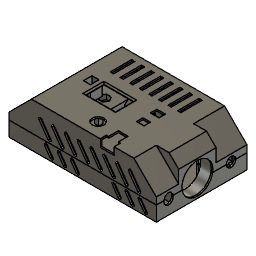
Arduino_Spot_Welder_V4_Case (Autodesk Fusion 360 design; units mm, degrees)
Autodesk Fusion 360 part; units mm, degrees
note: some values were not read from the file. Chosen so that the rebuilt part matches the saved one: a direction; which face or edge a step refers to; a side. Set by a fixed rule: which sketch regions a step uses.
(part 1 of 2)
sketch "Skizze1" plane through (0, 0, 0) normal (0, 1, 0) x (1, 0, 0)
  line L0 (-67.5, -41) -> (67.5, -41)
  line L1 (67.5, -41) -> (67.5, 41)
  line L2 (67.5, 41) -> (-67.5, 41)
  line L3 (-67.5, 41) -> (-67.5, -41)
  line L4 (1.75, 0) -> (22.5, 0)
  line L5 (0, -1.75) -> (0, -22.5)
  dimension "d1" = 82
  dimension "d2" = 135
  constraint horizontal L0
  constraint vertical L1
  constraint horizontal L2
  constraint vertical L3
  constraint symmetric L0 L2 L4
  constraint symmetric L1 L3 L5
  measures "d1" distance of L0.start L2.end
  measures "d2" distance of L0.start L0.end
extrude "Extrusion1" add sketch "Skizze1" along normal blind 1.5 makes body 1
sketch "Skizze2" plane through (0, 1.5, 0) normal (0, 1, 0) x (-1, 0, 0)
  line L0 (67.5, -41) -> (67.5, 41)
  line L1 (67.5, 41) -> (-67.5, 41)
  line L2 (-67.5, 41) -> (-67.5, -41)
  line L3 (-67.5, -41) -> (67.5, -41)
  line L4 (38.5, 39) -> (-38.5, 39)
  line L5 (-38.5, 39) -> (-38.5, -11)
  line L6 (-38.5, -11) -> (38.5, -11)
  line L7 (38.5, -11) -> (38.5, 39)
  line L8 (-1.75, 0) -> (-22.5, 0)
  line L9 (0, 1.75) -> (0, 22.5)
  circle A0 centre (35.5, 36) radius 1.65
  circle A1 centre (-35.5, -8) radius 1.65
  line L10 (38.5, 39) -> (32.5, 39)
  line L11 (32.5, 39) -> (32.5, 33)
  line L12 (32.5, 33) -> (38.5, 33)
  line L13 (38.5, 33) -> (38.5, 39)
  line L14 (-38.5, -11) -> (-32.5, -11)
  line L15 (-32.5, -11) -> (-32.5, -5)
  line L16 (-32.5, -5) -> (-38.5, -5)
  line L17 (-38.5, -5) -> (-38.5, -11)
  line L18 (38.5, -11) -> (34.5, -11)
  line L19 (34.5, -11) -> (34.5, -7)
  line L20 (34.5, -7) -> (38.5, -7)
  line L21 (38.5, -7) -> (38.5, -11)
  line L22 (-38.5, 39) -> (-34.5, 39)
  line L23 (-34.5, 39) -> (-34.5, 35)
  line L24 (-34.5, 35) -> (-38.5, 35)
  line L25 (-38.5, 35) -> (-38.5, 39)
  dimension "d5" = 77
  dimension "d6" = 50
  dimension "d7" = 2
  dimension "d8" = 3.3
  dimension "d9" = 3.3
  dimension "d10" = 3
  dimension "d11" = 3
  dimension "d12" = 3
  dimension "d13" = 3
  dimension "d14" = 6
  dimension "d15" = 6
  dimension "d16" = 6
  dimension "d17" = 6
  dimension "d302" = 4
  dimension "d303" = 4
  dimension "d304" = 4
  dimension "d305" = 4
  constraint horizontal L4
  constraint vertical L5
  constraint horizontal L6
  constraint vertical L7
  constraint symmetric L5 L7 L9
  constraint horizontal L10
  constraint vertical L11
  constraint horizontal L12
  constraint vertical L13
  constraint horizontal L14
  constraint vertical L15
  constraint horizontal L16
  constraint vertical L17
  constraint horizontal L18
  constraint vertical L19
  constraint horizontal L20
  constraint vertical L21
  constraint horizontal L22
  constraint vertical L23
  constraint horizontal L24
  constraint vertical L25
  measures "d5" distance of L4.start L4.end
  measures "d6" distance of L4.start L6.end
  measures "d7" distance of L1 L4
  measures "d8" diameter of A0
  measures "d9" diameter of A1
  measures "d10" distance of L4 A0.centre
  measures "d11" distance of L7 A0.centre
  measures "d12" distance of L5 A1.centre
  measures "d13" distance of L6 A1.centre
  measures "d14" distance of L4.start L10.end
  measures "d15" distance of L4.start L12.end
  measures "d16" distance of L5.end L14.end
  measures "d17" distance of L5.end L16.end
  measures "d302" distance of L6.end L18.end
  measures "d303" distance of L6.end L20.end
  measures "d304" distance of L4.end L22.end
  measures "d305" distance of L4.end L24.end
extrude "Extrusion2" add sketch "Skizze2" along normal blind 5.5 contours L4 L7 L10 L11 L12 L13 | L5 L6 L14 L15 L16 L17 bodies 1
extrude "Extrusion3" add 2 faces at (-35.3776, 1.5, 36.5362) (35.9032, 1.5, -8.3741) along direction (0, 1, 0) blind 2 on bodies 1 bodies 1
extrude "Extrusion57" add sketch "Skizze2" along normal blind 8 contours L4 L5 L22 L23 L24 L25 | L6 L7 L18 L19 L20 L21 bodies 1
sketch "Skizze3" plane through (0, 1.5, 0) normal (0, 1, 0) x (-1, 0, 0)
  line L0 (38.5, 33) -> (32.5, 33)
  line L1 (32.5, 33) -> (32.5, 39)
  line L2 (32.5, 39) -> (38.5, 39)
  line L3 (38.5, 39) -> (38.5, 33)
  line L4 (67.5, -41) -> (67.5, 41)
  line L5 (67.5, 41) -> (-67.5, 41)
  line L6 (-67.5, 41) -> (-67.5, -41)
  line L7 (-67.5, -41) -> (67.5, -41)
  line L8 (-38.5, -5) -> (-32.5, -5)
  line L9 (-32.5, -5) -> (-32.5, -11)
  line L10 (-32.5, -11) -> (-38.5, -11)
  line L11 (-38.5, -11) -> (-38.5, -5)
  line L12 (61, -16) -> (-25, -16)
  line L13 (-25, -16) -> (-25, -39)
  line L14 (-25, -39) -> (61, -39)
  line L15 (61, -39) -> (61, -16)
  line L16 (0, 1.75) -> (0, 22.5)
  line L17 (-1.75, 0) -> (-22.5, 0)
  line L18 (35.5, -39) -> (0.5, -39)
  line L19 (0.5, -39) -> (0.5, -16)
  line L20 (0.5, -16) -> (35.5, -16)
  line L21 (35.5, -16) -> (35.5, -39)
  line L22 (-38.5, 35) -> (-38.5, 39)
  line L23 (-38.5, 39) -> (-34.5, 39)
  line L24 (-34.5, 39) -> (-34.5, 35)
  line L25 (-34.5, 35) -> (-38.5, 35)
  line L26 (38.5, -7) -> (38.5, -11)
  line L27 (38.5, -11) -> (34.5, -11)
  line L28 (34.5, -11) -> (34.5, -7)
  line L29 (34.5, -7) -> (38.5, -7)
  dimension "d22" = 86
  dimension "d23" = 23
  dimension "d24" = 2
  dimension "d25" = 35
  dimension "d369" = 25.5
  dimension "d370" = 6.5
  constraint horizontal L12
  constraint vertical L13
  constraint horizontal L14
  constraint vertical L15
  constraint horizontal L18
  constraint vertical L19
  constraint horizontal L20
  constraint vertical L21
  constraint coincident L14 L18.start
  constraint collinear L12 L20
  measures "d22" distance of L12.start L12.end
  measures "d23" distance of L12.start L14.end
  measures "d24" distance of L7 L14
  measures "d25" distance of L18.start L18.end
  measures "d229" distance of L20.end
  measures "d369" distance of L13 L19
  measures "d370" distance of L4 L15
extrude "Extrusion4" add sketch "Skizze3" along normal blind 5 contours L12 L14 L15 L21 | L12 L13 L14 L19 bodies 1
sketch "Skizze4" plane through (0, 6.5, 0) normal (0, 1, 0) x (-1, 0, 0)
  line L0 (35.5, -16) -> (35.5, -39)
  line L1 (35.5, -39) -> (61, -39)
  line L2 (61, -39) -> (61, -16)
  line L3 (61, -16) -> (35.5, -16)
  line L4 (51.8383, -31.55) -> (54.1765, -27.5)
  line L5 (54.1765, -27.5) -> (51.8383, -23.45)
  line L6 (51.8383, -23.45) -> (47.1617, -23.45)
  line L7 (47.1617, -23.45) -> (44.8235, -27.5)
  line L8 (44.8235, -27.5) -> (47.1617, -31.55)
  line L9 (47.1617, -31.55) -> (51.8383, -31.55)
  line L10 (0, 1.75) -> (0, 22.5)
  circle A0 centre (49.5, -27.5) radius 2.6
  circle A1 centre (-13.5, -28) radius 2.6
  line L11 (-11.1617, -32.05) -> (-8.8235, -28)
  line L12 (-8.8235, -28) -> (-11.1617, -23.95)
  line L13 (-11.1617, -23.95) -> (-15.8383, -23.95)
  line L14 (-15.8383, -23.95) -> (-18.1765, -28)
  line L15 (-18.1765, -28) -> (-15.8383, -32.05)
  line L16 (-15.8383, -32.05) -> (-11.1617, -32.05)
  line L17 (0.5, -39) -> (0.5, -16)
  line L18 (-25, -39) -> (0.5, -39)
  point P0 (49.5, -27.5)
  point P1 (-13.5, -28)
  dimension "d28" = 4.05
  dimension "d29" = 11.5
  dimension "d31" = 14
  dimension "d35" = 5.2
  dimension "d371" = 5.2
  dimension "d372" = 4.05
  dimension "d373" = 14
  dimension "d374" = 11
  constraint parallel L1 L9
  constraint coincident P0 A0.centre
  constraint coincident P1 A1.centre
  constraint parallel L16 L18
  measures "d28" distance of P0 L9
  measures "d29" distance of L1 P0
  measures "d31" distance of L0 P0
  measures "d35" diameter of A0
  measures "d371" diameter of A1
  measures "d372" distance of P1 L16
  measures "d373" distance of P1 L17
  measures "d374" distance of P1 L18
extrude "Extrusion5" cut sketch "Skizze4" against normal blind 4.5 contours L4 L5 L6 L7 L8 L9 | A0 | A1 | L11 L12 L13 L14 L15 L16 bodies 1
extrude "Extrusion6" cut sketch "Skizze4" against normal up to surface (5.5 mm away) contours A0 | A1 bodies 1
sketch "Skizze6" plane through (0, 0, 0) normal (0, -1, 0) x (1, 0, 0)
  line L0 (-67.5, 41) -> (-67.5, -41)
  line L1 (-67.5, -41) -> (67.5, -41)
  line L2 (67.5, -41) -> (67.5, 41)
  line L3 (67.5, 41) -> (-67.5, 41)
  line L4 (-69, -42.5) -> (69, -42.5)
  line L5 (69, -42.5) -> (69, 42.5)
  line L6 (69, 42.5) -> (-69, 42.5)
  line L7 (-69, 42.5) -> (-69, -42.5)
  dimension "d38" = 1.5
  dimension "d39" = 1.5
  dimension "d40" = 1.5
  dimension "d41" = 1.5
  constraint horizontal L4
  constraint vertical L5
  constraint horizontal L6
  constraint vertical L7
  measures "d38" distance of L0 L7
  measures "d39" distance of L2 L5
  measures "d40" distance of L3 L6
  measures "d41" distance of L1 L4
extrude "Extrusion7" add sketch "Skizze6" against normal blind 14 bodies 1
extrude "Extrusion69" add 1 faces at (-36.5, 3.3333, 39) along direction (0, 0, 1) up to surface (2 mm away) on bodies 1 bodies 1
extrude "Extrusion71" add 1 faces at (35.8333, 4.1667, 39) along direction (0, 0, 1) up to surface (2 mm away) on bodies 1 bodies 1
sketch "Skizze58" plane through (0, 0, -11) normal (0, 0, -1) x (-1, 0, 0)
  line L0 (34.5, 1.5) -> (38.5, 1.5)
  line L1 (38.5, 1.5) -> (38.5, 9.5)
  line L2 (38.5, 9.5) -> (34.5, 9.5)
  line L3 (34.5, 9.5) -> (34.5, 1.5)
  line L4 (61, 1.5) -> (35.5, 1.5)
  line L5 (35.5, 1.5) -> (35.5, 6.5)
  line L6 (35.5, 6.5) -> (61, 6.5)
  line L7 (61, 6.5) -> (61, 1.5)
extrude "Extrusion73" add sketch "Skizze58" along normal up to surface (5 mm away) contours L0 L1 L4 L5 L6 bodies 1
sketch "Skizze7" plane through (-69, 0, 0) normal (-1, 0, 0) x (0, 0, 1)
  line L0 (-42.5, 0) -> (42.5, 0)
  line L1 (42.5, 0) -> (42.5, 14)
  line L2 (42.5, 14) -> (-42.5, 14)
  line L3 (-42.5, 14) -> (-42.5, 0)
  circle A0 centre (-27.5, 14) radius 4.5
  dimension "d44" = 9
  dimension "d46" = 15
  constraint coincident L2 A0.centre
  measures "d44" diameter of A0
  measures "d46" distance of L3 A0.centre
extrude "Extrusion8" cut sketch "Skizze7" against normal blind 138 contours L2 A0 picked at (-26.2064, 11.6926) bodies 1
sketch "Skizze8" plane through (-69, 0, 0) normal (-1, 0, 0) x (0, 0, 1)
  arc A0 (-32, 14) -> (-23, 14) centre (-27.5, 14) ccw
  line L0 (-32, 14) -> (-42.5, 14)
  line L1 (-42.5, 14) -> (-42.5, 0)
  line L2 (-42.5, 0) -> (42.5, 0)
  line L3 (42.5, 0) -> (42.5, 14)
  line L4 (42.5, 14) -> (-23, 14)
  circle A1 centre (-2.5, 14) radius 4.5
  dimension "d49" = 9
  dimension "d51" = 45
  constraint coincident L4 A1.centre
  measures "d49" diameter of A1
  measures "d51" distance of L3 A1.centre
extrude "Extrusion9" cut sketch "Skizze8" against normal blind 2 contours L4 A1 picked at (-1, 11.9595) bodies 1
sketch "Skizze9" plane through (69, 0, 0) normal (1, 0, 0) x (0, 0, -1)
  arc A0 (23, 14) -> (32, 14) centre (27.5, 14) ccw
  line L0 (23, 14) -> (-42.5, 14)
  line L1 (-42.5, 14) -> (-42.5, 0)
  line L2 (-42.5, 0) -> (42.5, 0)
  line L3 (42.5, 0) -> (42.5, 14)
  line L4 (42.5, 14) -> (32, 14)
  circle A1 centre (-31, 14) radius 4.25
  dimension "d54" = 8.5
  dimension "d55" = 11.5
  constraint coincident L0 A1.centre
  measures "d54" diameter of A1
  measures "d55" distance of L1 A1.centre
extrude "Extrusion10" cut sketch "Skizze9" against normal blind 2 contours L0 A1 picked at (-30.1084, 11.5575) bodies 1
extrude "Extrusion11" add 2 faces at (-44, 3.1667, -39) (16.5, 3.1667, -39) along direction (0, 0, -1) blind 2 on bodies 1 bodies 1
sketch "Skizze10" plane through (0, 14, 0) normal (0, 1, 0) x (-1, 0, 0)
  line L0 (-67.5, -32) -> (-69, -32)
  line L1 (-69, -32) -> (-69, -42.5)
  line L2 (-69, -42.5) -> (69, -42.5)
  line L3 (69, -42.5) -> (69, -32)
  line L4 (69, -32) -> (67.5, -32)
  line L5 (67.5, -32) -> (67.5, -41)
  line L6 (67.5, -41) -> (-67.5, -41)
  line L7 (-67.5, -41) -> (-67.5, -32)
  line L8 (-69, 35.25) -> (-67.5, 35.25)
  line L9 (-67.5, 35.25) -> (-67.5, 41)
  line L10 (-67.5, 41) -> (67.5, 41)
  line L11 (67.5, 41) -> (67.5, 2)
  line L12 (67.5, 2) -> (69, 2)
  line L13 (69, 2) -> (69, 42.5)
  line L14 (69, 42.5) -> (-69, 42.5)
  line L15 (-69, 42.5) -> (-69, 35.25)
  line L16 (-69, -42.5) -> (69, -42.5)
  line L17 (69, -42.5) -> (-69, -42.5)
  line L18 (-69, -42.5) -> (-69, 42.5)
  line L19 (-69, 42.5) -> (69, 42.5)
  line L20 (69, 42.5) -> (69, -42.5)
  line L21 (67.5, -41) -> (-67.5, -41)
  line L22 (-67.5, -41) -> (-67.5, 41)
  line L23 (-67.5, 41) -> (67.5, 41)
  line L24 (67.5, 41) -> (67.5, -41)
  constraint horizontal L17
  constraint vertical L18
  constraint horizontal L19
  constraint vertical L20
  constraint coincident L14.end L15.start
  constraint coincident L2.end L3.start
  constraint horizontal L21
  constraint vertical L22
  constraint horizontal L23
  constraint vertical L24
  constraint coincident L9.end L10.start
  constraint coincident L5.end L6.start
extrude "Extrusion12" add sketch "Skizze10" along normal blind 26 separate body contours L0 L1 L2 L3 L4 L5 L6 L7 L16 L17 L18 L20 L21 L22 L24 | L0 L8 L18 L22 | L8 L9 L10 L11 L12 L13 L14 L15 L18 L19 L20 L22 L23 L24 | L4 L12 L20 L24 makes body 2
sketch "Skizze11" plane through (0, 40, 0) normal (0, 1, 0) x (-1, 0, 0)
  line L0 (-67.5, 41) -> (67.5, 41)
  line L1 (67.5, 41) -> (67.5, -41)
  line L2 (67.5, -41) -> (-67.5, -41)
  line L3 (-67.5, -41) -> (-67.5, 41)
  line L4 (69, 42.5) -> (-69, 42.5)
  line L5 (-69, 42.5) -> (-69, -42.5)
  line L6 (-69, -42.5) -> (69, -42.5)
  line L7 (69, -42.5) -> (69, 42.5)
  line L8 (69, -42.5) -> (-69, -42.5)
  line L9 (-69, -42.5) -> (-69, 42.5)
  line L10 (-69, 42.5) -> (69, 42.5)
  line L11 (69, 42.5) -> (69, -42.5)
  constraint horizontal L8
  constraint vertical L9
  constraint horizontal L10
  constraint vertical L11
  constraint coincident L4.end L5.start
  constraint coincident L6.end L7.start
extrude "Extrusion13" add sketch "Skizze11" along normal blind 1.5 contours L0 L1 L2 L3 | L4 L5 L6 L7 L8 L9 L10 L11 bodies 2
sketch "Skizze12" plane through (0, 41.5, 0) normal (0, 1, 0) x (-1, 0, 0)
  line L0 (69, 42.5) -> (-69, 42.5)
  line L1 (-69, 42.5) -> (-69, -42.5)
  line L2 (-69, -42.5) -> (69, -42.5)
  line L3 (69, -42.5) -> (69, 42.5)
  line L4 (-38.5, 39) -> (-38.5, -11)
  line L5 (38.5, 39) -> (-38.5, 39)
  line L6 (-18.5, 42.5) -> (-27.5, 42.5)
  line L7 (-27.5, 42.5) -> (-27.5, 27.5)
  line L8 (-27.5, 27.5) -> (-18.5, 27.5)
  line L9 (-18.5, 27.5) -> (-18.5, 42.5)
  line L10 (-38.5, -11) -> (38.5, -11)
  line L11 (38.5, -11) -> (38.5, 39)
  circle A0 centre (-1.5, 29.5) radius 5.5
  line L12 (27, 19.5) -> (-0.8, 19.5)
  line L13 (-0.8, 19.5) -> (-0.8, -9)
  line L14 (-0.8, -9) -> (27, -9)
  line L15 (27, -9) -> (27, 19.5)
  line L16 (27, -4.5) -> (-0.8, -4.5)
  line L17 (-0.8, -4.5) -> (-0.8, 12.5)
  line L18 (-0.8, 12.5) -> (27, 12.5)
  line L19 (27, 12.5) -> (27, -4.5)
  line L20 (39, 2.2) -> (33, 2.2)
  line L21 (33, 2.2) -> (33, -3.8)
  line L22 (33, -3.8) -> (39, -3.8)
  line L23 (39, -3.8) -> (39, 2.2)
  line L24 (40, 3.2) -> (32, 3.2)
  line L25 (32, 3.2) -> (32, -4.8)
  line L26 (32, -4.8) -> (40, -4.8)
  line L27 (40, -4.8) -> (40, 3.2)
  line L28 (-19, -2) -> (-27, -2)
  line L29 (-27, -2) -> (-27, -8)
  line L30 (-27, -8) -> (-19, -8)
  line L31 (-19, -8) -> (-19, -2)
  line L32 (-19.5, 11.5) -> (-26.5, 11.5)
  line L33 (-26.5, 11.5) -> (-26.5, 7.5)
  line L34 (-26.5, 7.5) -> (-19.5, 7.5)
  line L35 (-19.5, 7.5) -> (-19.5, 11.5)
  line L36 (-23, 27.5) -> (-23, -9) construction
  dimension "d64" = 11
  dimension "d65" = 9
  dimension "d66" = 15
  dimension "d67" = 11
  dimension "d68" = 37
  dimension "d70" = 27.8
  dimension "d71" = 28.5
  dimension "d72" = 2
  dimension "d73" = 37.7
  dimension "d74" = 17
  dimension "d75" = 4.5
  dimension "d77" = 7.2
  dimension "d78" = 6
  dimension "d79" = 6
  dimension "d80" = 1
  dimension "d81" = 1
  dimension "d82" = 1
  dimension "d83" = 1
  dimension "d86" = 8
  dimension "d87" = 6
  dimension "d92" = 3
  dimension "d301" = 9.5
  dimension "d365" = 0.5
  dimension "d366" = 7
  dimension "d367" = 4
  dimension "d368" = 27.5
  constraint horizontal L6
  constraint vertical L7
  constraint horizontal L8
  constraint vertical L9
  constraint coincident L0 L6.start
  constraint horizontal L12
  constraint vertical L13
  constraint horizontal L14
  constraint vertical L15
  constraint horizontal L16
  constraint vertical L17
  constraint horizontal L18
  constraint vertical L19
  constraint coincident L13 L17.end
  constraint coincident L15 L16.start
  constraint horizontal L20
  constraint vertical L21
  constraint horizontal L22
  constraint vertical L23
  constraint horizontal L24
  constraint vertical L25
  constraint horizontal L26
  constraint vertical L27
  constraint horizontal L28
  constraint vertical L29
  constraint horizontal L30
  constraint vertical L31
  constraint horizontal L32
  constraint vertical L33
  constraint horizontal L34
  constraint vertical L35
  constraint midpoint L8 L36.start
  constraint perpendicular L10 L36
  constraint symmetric L29 L31 L36
  constraint symmetric L33 L35 L36
  measures "d64" distance of L4 L7
  measures "d65" distance of L7.end L8.end
  measures "d66" distance of L6.start L8.end
  measures "d67" diameter of A0
  measures "d68" distance of L4 A0.centre
  measures "d70" distance of L12.start L12.end
  measures "d71" distance of L12.start L14.end
  measures "d72" distance of L10 L14
  measures "d73" distance of L4 L13
  measures "d74" distance of L16 L18
  measures "d75" distance of L14 L16
  measures "d77" distance of L10 L22
  measures "d78" distance of L20.start L20.end
  measures "d79" distance of L20.end L21.end
  measures "d80" distance of L22 L26
  measures "d81" distance of L21 L25
  measures "d82" distance of L20 L24
  measures "d83" distance of L23 L27
  measures "d86" distance of L28.start L28.end
  measures "d87" distance of L28.start L30.end
  measures "d92" distance of L10 L30
  measures "d301" distance of L5 A0.centre
  measures "d365" distance of L11 L23
  measures "d366" distance of L32.start L32.end
  measures "d367" distance of L32.start L34.end
  measures "d368" distance of L5 L32
extrude "Extrusion14" cut sketch "Skizze12" against normal blind 7 contours L0 L5 L6 L7 L9 | L5 L7 L8 L9 | L11 L20 L21 L22 L24 L25 L26 | L11 L20 L21 L22 | A0 | L13 L15 L16 L17 L18 L19 | L28 L29 L30 L31 | L32 L33 L34 L35 bodies 2
sketch "Skizze13" plane through (-69, 0, 0) normal (-1, 0, 0) x (0, 0, 1)
  line L0 (-42.5, 14) -> (42.5, 14)
  line L1 (42.5, 14) -> (42.5, 41.5)
  line L2 (42.5, 41.5) -> (-42.5, 41.5)
  line L3 (-42.5, 41.5) -> (-42.5, 14)
  arc A0 (-7, 14) -> (2, 14) centre (-2.5, 14) ccw
  line L4 (-7, 14) -> (-23, 14)
  arc A1 (-32, 14) -> (-23, 14) centre (-27.5, 14) ccw
  line L5 (-32, 14) -> (-42.5, 14)
  line L6 (-42.5, 14) -> (-42.5, 0)
  line L7 (-42.5, 0) -> (42.5, 0)
  line L8 (42.5, 0) -> (42.5, 14)
  line L9 (42.5, 14) -> (2, 14)
  circle A2 centre (-27.5, 14) radius 4.5
  circle A3 centre (-2.5, 14) radius 4.5
  constraint concentric A1 A2
  constraint coincident L4.end A2
  constraint concentric A0 A3
  constraint coincident A0.end A3
extrude "Extrusion15" cut sketch "Skizze13" against normal blind 2 contours L0 A2 | L0 A3 bodies 2
sketch "Skizze14" plane through (69, 0, 0) normal (1, 0, 0) x (0, 0, -1)
  line L0 (-42.5, 14) -> (42.5, 14)
  line L1 (42.5, 14) -> (42.5, 41.5)
  line L2 (42.5, 41.5) -> (-42.5, 41.5)
  line L3 (-42.5, 41.5) -> (-42.5, 14)
  arc A0 (-35.25, 14) -> (-26.75, 14) centre (-31, 14) ccw
  line L4 (-35.25, 14) -> (-42.5, 14)
  line L5 (-42.5, 14) -> (-42.5, 0)
  line L6 (-42.5, 0) -> (42.5, 0)
  line L7 (42.5, 0) -> (42.5, 14)
  line L8 (42.5, 14) -> (32, 14)
  arc A1 (23, 14) -> (32, 14) centre (27.5, 14) ccw
  line L9 (23, 14) -> (-26.75, 14)
  circle A2 centre (-31, 14) radius 4.25
  circle A3 centre (27.5, 14) radius 4.5
  constraint concentric A0 A2
  constraint coincident A0.end A2
  constraint concentric A1 A3
  constraint coincident L8.end A3
extrude "Extrusion16" cut sketch "Skizze14" against normal blind 2 contours L0 A2 | L0 A3 bodies 2
sketch "Skizze15" plane through (0, 14, 0) normal (0, -1, 0) x (1, 0, 0)
  line L0 (69, -32) -> (67.5, -32)
  line L1 (67.5, -32) -> (67.5, -41)
  line L2 (67.5, -41) -> (-67.5, -41)
  line L3 (-67.5, -41) -> (-67.5, -32)
  line L4 (-67.5, -32) -> (-69, -32)
  line L5 (-69, -32) -> (-69, -42.5)
  line L6 (-69, -42.5) -> (69, -42.5)
  line L7 (69, -42.5) -> (69, -32)
  line L8 (-24.5, -41) -> (-9.5, -41)
  line L9 (-9.5, -41) -> (-9.5, -21)
  line L10 (-9.5, -21) -> (-24.5, -21)
  line L11 (-24.5, -21) -> (-24.5, -41)
  line L12 (0, 1.75) -> (0, 22.5)
  line L13 (-9.5, -41) -> (-24.5, -41)
  line L14 (-24.5, -41) -> (-24.5, -42.5)
  line L15 (-24.5, -42.5) -> (-9.5, -42.5)
  line L16 (-9.5, -42.5) -> (-9.5, -41)
  dimension "d98" = 15
  dimension "d99" = 20
  dimension "d411" = 43
  constraint horizontal L8
  constraint vertical L9
  constraint horizontal L10
  constraint vertical L11
  constraint coincident L2 L8.start
  constraint horizontal L13
  constraint vertical L14
  constraint horizontal L15
  constraint vertical L16
  constraint coincident L6 L14.end
  constraint collinear L11 L14
  measures "d98" distance of L8.start L8.end
  measures "d99" distance of L8.start L10.end
  measures "d411" distance of L3 L11
extrude "Extrusion19" add sketch "Skizze15" against normal blind 22 contours L2 L8 L9 L10 L11 L13 bodies 2
chamfer "Fase3" distance 20 angle 45 1 edges at (-17, 36, -21) on bodies 2
chamfer "Fase4" distance 9 angle 45 1 edges at (69, 41.5, 0) measured on face at (55, 41.5, -0.6667) on bodies 2
chamfer "Fase5" distance 21 angle 45 1 edges at (-69, 41.5, 0) measured on face at (-2.7333, 41.5, -29.8333) on bodies 2
sketch "Skizze16" plane through (-44.75, 44.75, 0) normal (-0.707107, 0.707107, 0) x (0, 0, 1)
  line L0 (41, -6.7175) -> (41, -32.1734)
  line L1 (41, -32.1734) -> (-41, -32.1734)
  line L2 (-41, -32.1734) -> (-41, -6.7175)
  line L3 (-41, -6.7175) -> (41, -6.7175)
  line L4 (42.5, -34.2947) -> (42.5, -4.5962)
  line L5 (42.5, -4.5962) -> (-42.5, -4.5962)
  line L6 (-42.5, -4.5962) -> (-42.5, -34.2947)
  line L7 (-42.5, -34.2947) -> (42.5, -34.2947)
extrude "Extrusion20" add sketch "Skizze16" against normal blind 1.5 contours L0 L1 L2 L3 | L4 L5 L6 L7 bodies 2
sketch "Skizze17" plane through (50.75, 50.75, 0) normal (0.707107, 0.707107, 0) x (0, 0, -1)
  line L0 (41, -23.6881) -> (-41, -23.6881)
  line L1 (-41, -23.6881) -> (-41, -15.2028)
  line L2 (-41, -15.2028) -> (41, -15.2028)
  line L3 (41, -15.2028) -> (41, -23.6881)
  line L4 (42.5, -25.8094) -> (42.5, -13.0815)
  line L5 (42.5, -13.0815) -> (-42.5, -13.0815)
  line L6 (-42.5, -13.0815) -> (-42.5, -25.8094)
  line L7 (-42.5, -25.8094) -> (42.5, -25.8094)
extrude "Extrusion21" add sketch "Skizze17" against normal blind 1.5 contours L0 L1 L2 L3 | L4 L5 L6 L7 bodies 2
sketch "Skizze18" plane through (0, 41.5, 0) normal (0, 1, 0) x (-1, 0, 0)
  line L0 (48, -42.5) -> (48, 42.5)
  line L1 (48, 42.5) -> (-18.5, 42.5)
  line L2 (-18.5, 42.5) -> (-18.5, 27.5)
  line L3 (-18.5, 27.5) -> (-27.5, 27.5)
  line L4 (-27.5, 27.5) -> (-27.5, 42.5)
  line L5 (-27.5, 42.5) -> (-60, 42.5)
  line L6 (-60, 42.5) -> (-60, -42.5)
  line L7 (-60, -42.5) -> (48, -42.5)
  line L8 (-27, -2) -> (-19, -2)
  line L9 (-19, -2) -> (-19, -8)
  line L10 (-19, -8) -> (-27, -8)
  line L11 (-27, -8) -> (-27, -2)
  line L12 (-0.8, -4.5) -> (-0.8, 12.5)
  line L13 (-0.8, 12.5) -> (27, 12.5)
  line L14 (27, 12.5) -> (27, -4.5)
  line L15 (27, -4.5) -> (-0.8, -4.5)
  line L16 (38.5, 3.2) -> (38.5, -4.8)
  line L17 (38.5, -4.8) -> (32, -4.8)
  line L18 (32, -4.8) -> (32, 3.2)
  line L19 (32, 3.2) -> (38.5, 3.2)
  circle A0 centre (-1.5, 29.5) radius 5.5
  line L20 (-16.5, 42.5) -> (-29.5, 42.5)
  line L21 (-29.5, 42.5) -> (-29.5, 36.5)
  line L22 (-29.5, 36.5) -> (-16.5, 36.5)
  line L23 (-16.5, 36.5) -> (-16.5, 42.5)
  line L24 (-26.5, 11.5) -> (-19.5, 11.5)
  line L25 (-19.5, 11.5) -> (-19.5, 7.5)
  line L26 (-19.5, 7.5) -> (-26.5, 7.5)
  line L27 (-26.5, 7.5) -> (-26.5, 11.5)
  dimension "d117" = 2
  dimension "d118" = 2
  dimension "d119" = 6
  constraint horizontal L20
  constraint vertical L21
  constraint horizontal L22
  constraint vertical L23
  constraint coincident L1 L20.start
  measures "d117" distance of L2 L23
  measures "d118" distance of L4 L21
  measures "d119" distance of L20 L22
extrude "Extrusion22" cut sketch "Skizze18" against normal blind 7 contours L1 L2 L20 L22 L23 | L2 L4 L20 L22 | L4 L5 L20 L21 L22 bodies 2
sketch "Skizze19" plane through (0, 41.5, 0) normal (0, 1, 0) x (-1, 0, 0)
  line L0 (-29.5, 36.5) -> (-29.5, 42.5)
  line L1 (-29.5, 42.5) -> (-60, 42.5)
  line L2 (-60, 42.5) -> (-60, -42.5)
  line L3 (-60, -42.5) -> (48, -42.5)
  line L4 (48, -42.5) -> (48, 42.5)
  line L5 (48, 42.5) -> (-16.5, 42.5)
  line L6 (-16.5, 42.5) -> (-16.5, 36.5)
  line L7 (-16.5, 36.5) -> (-18.5, 36.5)
  line L8 (-18.5, 36.5) -> (-18.5, 27.5)
  line L9 (-18.5, 27.5) -> (-27.5, 27.5)
  line L10 (-27.5, 27.5) -> (-27.5, 36.5)
  line L11 (-27.5, 36.5) -> (-29.5, 36.5)
  line L12 (-27, -2) -> (-19, -2)
  line L13 (-19, -2) -> (-19, -8)
  line L14 (-19, -8) -> (-27, -8)
  line L15 (-27, -8) -> (-27, -2)
  line L16 (-0.8, -4.5) -> (-0.8, 12.5)
  line L17 (-0.8, 12.5) -> (27, 12.5)
  line L18 (27, 12.5) -> (27, -4.5)
  line L19 (27, -4.5) -> (-0.8, -4.5)
  line L20 (38.5, 3.2) -> (38.5, -4.8)
  line L21 (38.5, -4.8) -> (32, -4.8)
  line L22 (32, -4.8) -> (32, 3.2)
  line L23 (32, 3.2) -> (38.5, 3.2)
  circle A0 centre (-1.5, 29.5) radius 5.5
  line L24 (-38.5, 39) -> (-38.5, -11)
  line L25 (38.5, 39) -> (-38.5, 39)
  line L26 (33, -16.5) -> (30, -16.5)
  line L27 (30, -16.5) -> (30, -36.5)
  line L28 (30, -36.5) -> (33, -36.5)
  line L29 (33, -36.5) -> (33, -16.5)
  line L30 (0, 1.75) -> (0, 22.5)
  line L31 (24, -16.5) -> (21, -16.5)
  line L32 (21, -16.5) -> (21, -36.5)
  line L33 (21, -36.5) -> (24, -36.5)
  line L34 (24, -36.5) -> (24, -16.5)
  line L35 (15, -16.5) -> (12, -16.5)
  line L36 (12, -16.5) -> (12, -36.5)
  line L37 (12, -36.5) -> (15, -36.5)
  line L38 (15, -36.5) -> (15, -16.5)
  line L39 (6, -16.5) -> (3, -16.5)
  line L40 (3, -16.5) -> (3, -36.5)
  line L41 (3, -36.5) -> (6, -36.5)
  line L42 (6, -36.5) -> (6, -16.5)
  line L43 (-12, -16.5) -> (-12, -36.5)
  line L44 (-15, -36.5) -> (-15, -16.5)
  line L45 (-15, -16.5) -> (-12, -16.5)
  line L46 (-12, -36.5) -> (-15, -36.5)
  line L47 (-6, -16.5) -> (-3, -16.5)
  line L48 (-3, -16.5) -> (-3, -36.5)
  line L49 (-3, -36.5) -> (-6, -36.5)
  line L50 (-6, -36.5) -> (-6, -16.5)
  line L51 (-24, -36.5) -> (-24, -16.5)
  line L52 (-24, -16.5) -> (-21, -16.5)
  line L53 (-21, -36.5) -> (-24, -36.5)
  line L54 (-21, -16.5) -> (-21, -36.5)
  line L55 (-33, -36.5) -> (-33, -16.5)
  line L56 (-33, -16.5) -> (-30, -16.5)
  line L57 (-30, -36.5) -> (-33, -36.5)
  line L58 (-30, -16.5) -> (-30, -36.5)
  line L59 (-26.5, 11.5) -> (-19.5, 11.5)
  line L60 (-19.5, 11.5) -> (-19.5, 7.5)
  line L61 (-19.5, 7.5) -> (-26.5, 7.5)
  line L62 (-26.5, 7.5) -> (-26.5, 11.5)
  dimension "d126" = 20
  dimension "d127" = 3
  dimension "d128" = 20
  dimension "d129" = 3
  dimension "d130" = 3
  dimension "d131" = 20
  dimension "d132" = 3
  dimension "d133" = 20
  dimension "d134" = 6
  dimension "d135" = 3
  dimension "d136" = 6
  dimension "d137" = 6
  dimension "d138" = 6
  constraint horizontal L26
  constraint vertical L27
  constraint horizontal L28
  constraint vertical L29
  constraint horizontal L31
  constraint vertical L32
  constraint horizontal L33
  constraint vertical L34
  constraint horizontal L35
  constraint vertical L36
  constraint horizontal L37
  constraint vertical L38
  constraint horizontal L39
  constraint vertical L40
  constraint horizontal L41
  constraint vertical L42
  constraint collinear L28 L33
  constraint collinear L33 L37
  constraint collinear L37 L41
  constraint symmetric L26.start L30 L55.end
  constraint symmetric L26.end L30 L56.end
  constraint symmetric L27.end L30 L57.start
  constraint symmetric L28.end L30 L55.start
  constraint symmetric L30 L31.start L51.end
  constraint symmetric L30 L31.end L52.end
  constraint symmetric L30 L32.end L53.start
  constraint symmetric L30 L33.end L51.start
  constraint symmetric L30 L35.start L44.end
  constraint symmetric L30 L35.end L43.start
  constraint symmetric L30 L36.end L43.end
  constraint symmetric L30 L37.end L44.start
  constraint symmetric L30 L39.start L47.start
  constraint symmetric L30 L39.end L47.end
  constraint symmetric L30 L40.end L48.end
  constraint symmetric L30 L41.end L49.end
  measures "d126" distance of L26.end L27.end
  measures "d127" distance of L26.start L26.end
  measures "d128" distance of L31.end L32.end
  measures "d129" distance of L32.end L33.end
  measures "d130" distance of L36.end L37.end
  measures "d131" distance of L35.end L36.end
  measures "d132" distance of L39.start L39.end
  measures "d133" distance of L39.end L40.end
  measures "d134" distance of L3 L28
  measures "d135" distance of L30 L40
  measures "d136" distance of L36 L42
  measures "d137" distance of L32 L38
  measures "d138" distance of L27 L34
extrude "Extrusion23" cut sketch "Skizze19" against normal blind 1.5 contours L26 L27 L28 L29 | L31 L32 L33 L34 | L35 L36 L37 L38 | L39 L40 L41 L42 | L43 L44 L45 L46 | L47 L48 L49 L50 | L51 L52 L53 L54 | L55 L56 L57 L58 bodies 2
sketch "Skizze20" plane through (0, 0, -42.5) normal (0, 0, -1) x (-1, 0, 0)
  line L0 (-69, 32.5) -> (-69, 14)
  line L1 (-69, 14) -> (69, 14)
  line L2 (69, 14) -> (69, 20.5)
  line L3 (69, 20.5) -> (48, 41.5)
  line L4 (48, 41.5) -> (-60, 41.5)
  line L5 (-60, 41.5) -> (-69, 32.5)
  line L6 (0.5, 1.5) -> (-25, 1.5)
  line L7 (-25, 1.5) -> (-25, 6.5)
  line L8 (-25, 6.5) -> (0.5, 6.5)
  line L9 (0.5, 6.5) -> (0.5, 1.5)
  line L10 (61, 1.5) -> (38.5, 1.5)
  line L11 (38.5, 6.5) -> (61, 6.5)
  line L12 (61, 6.5) -> (61, 1.5)
  line L13 (4.5, 3.1) -> (34.5, 3.1)
  line L14 (34.5, 3.1) -> (34.5, 11)
  line L15 (34.5, 11) -> (4.5, 11)
  line L16 (4.5, 11) -> (4.5, 3.1)
  line L17 (-38.5, 1.5) -> (38.5, 1.5)
  line L18 (0, 1.75) -> (0, 22.5)
  line L19 (5.7287, 2.2396) -> (11.2604, 10.1396)
  arc A0 (11.2604, 10.1396) -> (8.8029, 11.8604) centre (10.0316, 11) ccw
  line L20 (8.8029, 11.8604) -> (3.2713, 3.9604)
  arc A1 (3.2713, 3.9604) -> (5.7287, 2.2396) centre (4.5, 3.1) ccw
  line L21 (4.5, 3.1) -> (10.0316, 11) construction
  line L22 (4.5, 3.1) -> (-1.9764, 3.1) construction
  line L23 (21.0029, 11.8604) -> (15.4713, 3.9604)
  line L24 (17.9287, 2.2396) -> (23.4604, 10.1396)
  arc A2 (23.4604, 10.1396) -> (21.0029, 11.8604) centre (22.2316, 11) ccw
  arc A3 (15.4713, 3.9604) -> (17.9287, 2.2396) centre (16.7, 3.1) ccw
  line L25 (33.2713, 11.8604) -> (27.7396, 3.9604)
  arc A4 (35.7287, 10.1396) -> (33.2713, 11.8604) centre (34.5, 11) ccw
  line L26 (30.1971, 2.2396) -> (35.7287, 10.1396)
  arc A5 (27.7396, 3.9604) -> (30.1971, 2.2396) centre (28.9684, 3.1) ccw
  line L27 (38.5, 1.5) -> (38.5, 6.5)
  line L28 (-29, 3.1) -> (-59, 3.1)
  line L29 (-59, 3.1) -> (-59, 11)
  line L30 (-59, 11) -> (-29, 11)
  line L31 (-29, 11) -> (-29, 3.1)
  line L32 (69, 0) -> (-69, 0)
  line L33 (-57.7713, 2.2396) -> (-52.2396, 10.1396)
  arc A6 (-52.2396, 10.1396) -> (-54.6971, 11.8604) centre (-53.4684, 11) ccw
  line L34 (-54.6971, 11.8604) -> (-60.2287, 3.9604)
  arc A7 (-60.2287, 3.9604) -> (-57.7713, 2.2396) centre (-59, 3.1) ccw
  line L35 (-59, 3.1) -> (-53.4684, 11) construction
  line L36 (-30.2287, 11.8604) -> (-35.7604, 3.9604)
  arc A8 (-35.7604, 3.9604) -> (-33.3029, 2.2396) centre (-34.5316, 3.1) ccw
  line L37 (-33.3029, 2.2396) -> (-27.7713, 10.1396)
  arc A9 (-27.7713, 10.1396) -> (-30.2287, 11.8604) centre (-29, 11) ccw
  line L38 (-29, 11) -> (-34.5316, 3.1) construction
  line L39 (-45.5713, 2.2396) -> (-40.0396, 10.1396)
  arc A10 (-40.0396, 10.1396) -> (-42.4971, 11.8604) centre (-41.2684, 11) ccw
  line L40 (-42.4971, 11.8604) -> (-48.0287, 3.9604)
  arc A11 (-48.0287, 3.9604) -> (-45.5713, 2.2396) centre (-46.8, 3.1) ccw
  line L41 (-46.8, 3.1) -> (-41.2684, 11) construction
  dimension "d142" = 3
  dimension "d145" = 55
  dimension "d146" = 3
  dimension "d148" = 3
  dimension "d150" = 3
  dimension "d155" = 55
  dimension "d156" = 55
  dimension "d392" = 30
  dimension "d393" = 1.6
  dimension "d395" = 12.2
  dimension "d396" = 4
  dimension "d397" = 30
  dimension "d398" = 3
  dimension "d400" = 1.6
  dimension "d401" = 29
  dimension "d402" = 3
  dimension "d403" = 55
  dimension "d404" = 3
  dimension "d405" = 55
  dimension "d406" = 3
  dimension "d407" = 55
  dimension "d408" = 12.2
  constraint horizontal L13
  constraint vertical L14
  constraint horizontal L15
  constraint vertical L16
  constraint tangent L19 A0
  constraint tangent A0 L20
  constraint parallel L19 L20
  constraint tangent L20 A1
  constraint tangent L19 A1
  constraint coincident L15 A0.centre
  constraint coincident L13.start L16.end
  constraint tangent L24 A2
  constraint tangent L23 A2
  constraint parallel L23 L24
  constraint tangent L23 A3
  constraint tangent L24 A3
  constraint tangent A4 L26
  constraint tangent L25 A4
  constraint parallel L25 L26
  constraint tangent L25 A5
  constraint tangent L26 A5
  constraint coincident L15 A2.centre
  constraint coincident L22 A3.centre
  constraint coincident L15 L14.end
  constraint coincident L13 A5.centre
  constraint coincident L14.end L15.start
  constraint coincident L13 A3.centre
  constraint horizontal L28
  constraint vertical L29
  constraint horizontal L30
  constraint vertical L31
  constraint tangent L33 A6
  constraint tangent A6 L34
  constraint parallel L33 L34
  constraint tangent L34 A7
  constraint tangent L33 A7
  constraint coincident L28.end L29.start
  constraint coincident L30 A6.centre
  constraint tangent L36 A8
  constraint tangent A8 L37
  constraint parallel L36 L37
  constraint tangent L37 A9
  constraint tangent L36 A9
  constraint coincident L30.end L31.start
  constraint coincident L28 A8.centre
  constraint tangent L39 A10
  constraint tangent A10 L40
  constraint parallel L39 L40
  constraint tangent L40 A11
  constraint tangent L39 A11
  constraint coincident L28 A11.centre
  constraint coincident L30 A10.centre
  measures "d142" distance of L1 L15
  measures "d145" angle of L21 L22
  measures "d146" diameter of A0
  measures "d148" diameter of A2
  measures "d150" diameter of A4
  measures "d155" angle of L13 L24
  measures "d156" angle of L13 L26
  measures "d392" distance of L13.start L13.end
  measures "d393" distance of L17 L22
  measures "d395" distance of L13.start A3.centre
  measures "d396" distance of L9 L16
  measures "d397" distance of L28.start L28.end
  measures "d398" distance of L1 L30
  measures "d400" distance of L17 L28
  measures "d401" distance of L18 L31
  measures "d402" diameter of A6
  measures "d403" angle of L28 L33
  measures "d404" diameter of A8
  measures "d405" angle of L28 L37
  measures "d406" diameter of A10
  measures "d407" angle of L28 L39
  measures "d408" distance of L28.end A11.centre
extrude "Extrusion25" cut sketch "Skizze20" against normal blind 1.5 contours L13 L15 L16 L19 A0 L20 | L13 L16 L19 L20 A1 | L13 L15 L23 L24 A2 A3 | L13 L24 A3 | L15 A0 L20 | L13 L14 L15 L25 L26 A5 | L13 L26 A5 | L15 L23 A2 | L14 L15 L25 A4 L26 | L28 A8 L37 | L28 L30 L31 L36 A8 L37 | L30 L31 L36 L37 A9 | L28 L39 A11 | L28 L30 L39 A10 L40 A11 | L30 A10 L40 | L28 L29 L33 L34 A7 | L28 L29 L30 L33 A6 L34 | L30 A6 L34 bodies 1
sketch "Skizze62" plane through (0, 0, 42.5) normal (0, 0, 1) x (1, 0, 0)
  line L0 (-69, 0) -> (69, 0)
  line L1 (69, 0) -> (69, 14)
  line L2 (69, 14) -> (-69, 14)
  line L3 (-69, 14) -> (-69, 0)
  line L4 (35.7604, 3.9604) -> (30.2287, 11.8604)
  arc A0 (30.2287, 11.8604) -> (27.7713, 10.1396) centre (29, 11) ccw
  line L5 (27.7713, 10.1396) -> (33.3029, 2.2396)
  arc A1 (33.3029, 2.2396) -> (35.7604, 3.9604) centre (34.5316, 3.1) ccw
  line L6 (-11.2604, 10.1396) -> (-5.7287, 2.2396)
  arc A2 (-5.7287, 2.2396) -> (-3.2713, 3.9604) centre (-4.5, 3.1) ccw
  line L7 (-3.2713, 3.9604) -> (-8.8029, 11.8604)
  arc A3 (-8.8029, 11.8604) -> (-11.2604, 10.1396) centre (-10.0316, 11) ccw
  line L8 (40.0396, 10.1396) -> (45.5713, 2.2396)
  arc A4 (45.5713, 2.2396) -> (48.0287, 3.9604) centre (46.8, 3.1) ccw
  line L9 (48.0287, 3.9604) -> (42.4971, 11.8604)
  arc A5 (42.4971, 11.8604) -> (40.0396, 10.1396) centre (41.2684, 11) ccw
  line L10 (-35.7287, 10.1396) -> (-30.1971, 2.2396)
  arc A6 (-30.1971, 2.2396) -> (-27.7396, 3.9604) centre (-28.9684, 3.1) ccw
  line L11 (-27.7396, 3.9604) -> (-33.2713, 11.8604)
  arc A7 (-33.2713, 11.8604) -> (-35.7287, 10.1396) centre (-34.5, 11) ccw
  line L12 (-23.4604, 10.1396) -> (-17.9287, 2.2396)
  arc A8 (-17.9287, 2.2396) -> (-15.4713, 3.9604) centre (-16.7, 3.1) ccw
  line L13 (-15.4713, 3.9604) -> (-21.0029, 11.8604)
  arc A9 (-21.0029, 11.8604) -> (-23.4604, 10.1396) centre (-22.2316, 11) ccw
  line L14 (52.2396, 10.1396) -> (57.7713, 2.2396)
  arc A10 (57.7713, 2.2396) -> (60.2287, 3.9604) centre (59, 3.1) ccw
  line L15 (60.2287, 3.9604) -> (54.6971, 11.8604)
  arc A11 (54.6971, 11.8604) -> (52.2396, 10.1396) centre (53.4684, 11) ccw
  line L16 (69, 0) -> (-69, 0)
  line L17 (-69, 0) -> (-69, 14)
  line L18 (-69, 14) -> (69, 14)
  line L19 (69, 14) -> (69, 0)
extrude "Extrusion77" cut sketch "Skizze62" against normal up to surface (1.5 mm away) contours L4 A0 L5 A1 | L6 A2 L7 A3 | L8 A4 L9 A5 | L10 A6 L11 A7 | L12 A8 L13 A9 | L14 A10 L15 A11 bodies 1
sketch "Skizze21" plane through (0, 0, -42.5) normal (0, 0, -1) x (-1, 0, 0)
  line L0 (-69, 32.5) -> (-69, 14)
  line L1 (-69, 14) -> (69, 14)
  line L2 (69, 14) -> (69, 20.5)
  line L3 (69, 20.5) -> (48, 41.5)
  line L4 (48, 41.5) -> (-60, 41.5)
  line L5 (-60, 41.5) -> (-69, 32.5)
  line L6 (-34.1677, 17.1396) -> (-24.4169, 31.0652)
  arc A0 (-24.4169, 31.0652) -> (-26.8743, 32.7859) centre (-25.6456, 31.9256) ccw
  line L7 (-26.8743, 32.7859) -> (-36.6251, 18.8604)
  arc A1 (-36.6251, 18.8604) -> (-34.1677, 17.1396) centre (-35.3964, 18) ccw
  line L8 (-35.3964, 18) -> (-25.6456, 31.9256) construction
  line L9 (-14.6595, 32.7859) -> (-24.4103, 18.8604)
  arc A2 (-12.202, 31.0652) -> (-14.6595, 32.7859) centre (-13.4308, 31.9256) ccw
  line L10 (-21.9528, 17.1396) -> (-12.202, 31.0652)
  arc A3 (-24.4103, 18.8604) -> (-21.9528, 17.1396) centre (-23.1816, 18) ccw
  line L11 (-10.0358, 17.1396) -> (-0.285, 31.0652)
  line L12 (-11.2645, 18) -> (-1.5137, 31.9256) construction
  arc A4 (-12.4933, 18.8604) -> (-10.0358, 17.1396) centre (-11.2645, 18) ccw
  line L13 (9.3018, 32.7859) -> (-0.449, 18.8604)
  line L14 (-2.7425, 32.7859) -> (-12.4933, 18.8604)
  arc A5 (11.7592, 31.0652) -> (9.3018, 32.7859) centre (10.5305, 31.9256) ccw
  line L15 (2.0084, 17.1396) -> (11.7592, 31.0652)
  arc A6 (-0.285, 31.0652) -> (-2.7425, 32.7859) centre (-1.5137, 31.9256) ccw
  arc A7 (-0.449, 18.8604) -> (2.0084, 17.1396) centre (0.7797, 18) ccw
  arc A8 (23.6878, 18.8604) -> (26.1453, 17.1396) centre (24.9166, 18) ccw
  line L16 (20.978, 32.7859) -> (11.2272, 18.8604)
  line L17 (12.4559, 18) -> (22.2067, 31.9256) construction
  arc A9 (35.8961, 31.0652) -> (33.4386, 32.7859) centre (34.6674, 31.9256) ccw
  arc A10 (23.4355, 31.0652) -> (20.978, 32.7859) centre (22.2067, 31.9256) ccw
  line L18 (33.4386, 32.7859) -> (23.6878, 18.8604)
  arc A11 (11.2272, 18.8604) -> (13.6847, 17.1396) centre (12.4559, 18) ccw
  line L19 (26.1453, 17.1396) -> (35.8961, 31.0652)
  line L20 (13.6847, 17.1396) -> (23.4355, 31.0652)
  line L21 (-37.5876, 14) -> (32.0368, 14)
  line L22 (32.0368, 14) -> (32.0368, 18)
  line L23 (32.0368, 18) -> (-37.5876, 18)
  line L24 (-37.5876, 18) -> (-37.5876, 14)
  dimension "d157" = 3
  dimension "d158" = 3
  dimension "d159" = 3
  dimension "d160" = 3
  dimension "d161" = 3
  dimension "d162" = 3
  dimension "d163" = 55
  dimension "d166" = 4
  dimension "d167" = 17
  constraint tangent L6 A0
  constraint tangent A0 L7
  constraint parallel L6 L7
  constraint tangent L7 A1
  constraint tangent L6 A1
  constraint tangent A2 L10
  constraint tangent L9 A2
  constraint parallel L9 L10
  constraint tangent L9 A3
  constraint tangent L10 A3
  constraint tangent L11 A6
  constraint tangent L14 A6
  constraint parallel L11 L14
  constraint tangent A4 L14
  constraint tangent L11 A4
  constraint tangent A5 L15
  constraint tangent L13 A5
  constraint parallel L13 L15
  constraint tangent L13 A7
  constraint tangent L15 A7
  constraint tangent A10 L20
  constraint tangent L16 A10
  constraint parallel L16 L20
  constraint tangent L16 A11
  constraint tangent A11 L20
  constraint tangent A9 L19
  constraint tangent A9 L18
  constraint parallel L18 L19
  constraint tangent A8 L18
  constraint tangent A8 L19
  constraint parallel L6 L9
  constraint parallel L10 L14
  constraint parallel L11 L13
  constraint parallel L15 L16
  constraint parallel L18 L20
  constraint horizontal L21
  constraint vertical L22
  constraint horizontal L23
  constraint vertical L24
  constraint coincident L1 L21.start
  constraint coincident A1.centre L23
  constraint coincident A3.centre L23
  constraint coincident L12.start L23
  constraint coincident A7.centre L23
  constraint coincident L17.start L23
  constraint coincident A8.centre L23
  constraint equal L6 L9
  constraint equal L10 L14
  constraint equal L11 L13
  constraint equal L15 L16
  constraint equal L18 L20
  measures "d157" diameter of A0
  measures "d158" diameter of A2
  measures "d159" diameter of A6
  measures "d160" diameter of A5
  measures "d161" diameter of A10
  measures "d162" diameter of A9
  measures "d163" angle of L1 L6
  measures "d166" distance of L21 L23
  measures "d167" distance of A1.centre A0.centre
extrude "Extrusion26" cut sketch "Skizze21" against normal blind 1.5 contours L6 A1 L23 | L6 A0 L7 A1 L23 | A8 A9 L18 L19 L23 | A8 L19 L23 | L10 A3 L23 | L9 A2 L10 A3 L23 | L16 A10 A11 L20 L23 | A11 L20 L23 | L11 A4 L23 | L11 A4 L14 A6 L23 | L13 A5 L15 A7 L23 | L15 A7 L23 bodies 2
sketch "Skizze22" plane through (0, 40, 0) normal (0, -1, 0) x (1, 0, 0)
  line L0 (12, -16.5) -> (15, -16.5)
  line L1 (15, -16.5) -> (15, -36.5)
  line L2 (15, -36.5) -> (12, -36.5)
  line L3 (12, -36.5) -> (12, -16.5)
  line L4 (-24, -16.5) -> (-21, -16.5)
  line L5 (-21, -16.5) -> (-21, -36.5)
  line L6 (-21, -36.5) -> (-24, -36.5)
  line L7 (-24, -36.5) -> (-24, -16.5)
  line L8 (-15, -16.5) -> (-12, -16.5)
  line L9 (-12, -16.5) -> (-12, -36.5)
  line L10 (-12, -36.5) -> (-15, -36.5)
  line L11 (-15, -36.5) -> (-15, -16.5)
  line L12 (24, -16.5) -> (24, -36.5)
  line L13 (24, -36.5) -> (21, -36.5)
  line L14 (21, -36.5) -> (21, -16.5)
  line L15 (21, -16.5) -> (24, -16.5)
  line L16 (3, -36.5) -> (3, -16.5)
  line L17 (3, -16.5) -> (6, -16.5)
  line L18 (6, -16.5) -> (6, -36.5)
  line L19 (6, -36.5) -> (3, -36.5)
  line L20 (-33, -16.5) -> (-30, -16.5)
  line L21 (-30, -16.5) -> (-30, -36.5)
  line L22 (-30, -36.5) -> (-33, -36.5)
  line L23 (-33, -36.5) -> (-33, -16.5)
  line L24 (-6, -16.5) -> (-3, -16.5)
  line L25 (-3, -16.5) -> (-3, -36.5)
  line L26 (-3, -36.5) -> (-6, -36.5)
  line L27 (-6, -36.5) -> (-6, -16.5)
  line L28 (33, -16.5) -> (33, -36.5)
  line L29 (33, -36.5) -> (30, -36.5)
  line L30 (30, -36.5) -> (30, -16.5)
  line L31 (30, -16.5) -> (33, -16.5)
  circle A0 centre (1.5, 29.5) radius 5.5
  line L32 (-38.5, -4.8) -> (-38.5, 3.2)
  line L33 (-38.5, 3.2) -> (-32, 3.2)
  line L34 (-32, 3.2) -> (-32, -4.8)
  line L35 (-32, -4.8) -> (-38.5, -4.8)
  line L36 (0.8, 12.5) -> (0.8, -4.5)
  line L37 (0.8, -4.5) -> (-27, -4.5)
  line L38 (-27, -4.5) -> (-27, 12.5)
  line L39 (-27, 12.5) -> (0.8, 12.5)
  line L40 (19, -2) -> (27, -2)
  line L41 (27, -2) -> (27, -8)
  line L42 (27, -8) -> (19, -8)
  line L43 (19, -8) -> (19, -2)
  line L44 (29.5, 41) -> (29.5, 36.5)
  line L45 (29.5, 36.5) -> (27.5, 36.5)
  line L46 (27.5, 36.5) -> (27.5, 27.5)
  line L47 (27.5, 27.5) -> (18.5, 27.5)
  line L48 (18.5, 27.5) -> (18.5, 36.5)
  line L49 (18.5, 36.5) -> (16.5, 36.5)
  line L50 (16.5, 36.5) -> (16.5, 41)
  line L51 (16.5, 41) -> (-47.3787, 41)
  line L52 (-47.3787, 41) -> (-47.3787, -41)
  line L53 (-47.3787, -41) -> (59.3787, -41)
  line L54 (59.3787, -41) -> (59.3787, 41)
  line L55 (59.3787, 41) -> (29.5, 41)
  line L56 (-40, -6.3) -> (-30.5, -6.3)
  line L57 (-30.5, -6.3) -> (-30.5, 4.7)
  line L58 (-30.5, 4.7) -> (-40, 4.7)
  line L59 (-40, 4.7) -> (-40, -6.3)
  line L60 (19.5, 11.5) -> (26.5, 11.5)
  line L61 (26.5, 11.5) -> (26.5, 7.5)
  line L62 (26.5, 7.5) -> (19.5, 7.5)
  line L63 (19.5, 7.5) -> (19.5, 11.5)
  dimension "d169" = 1.5
  dimension "d170" = 1.5
  dimension "d171" = 1.5
  dimension "d172" = 1.5
  constraint horizontal L56
  constraint vertical L57
  constraint horizontal L58
  constraint vertical L59
  measures "d169" distance of L33 L58
  measures "d170" distance of L34 L57
  measures "d171" distance of L35 L56
  measures "d172" distance of L32 L59
extrude "Extrusion27" add sketch "Skizze22" along normal blind 12 contours L56 L57 L58 L59 bodies 2
sketch "Skizze23" plane through (0, 1.5, 0) normal (0, 1, 0) x (-1, 0, 0)
  line L0 (0.5, -16) -> (0.5, -41)
  line L1 (0.5, -41) -> (35.5, -41)
  line L2 (35.5, -41) -> (35.5, -11)
  line L3 (61, -16) -> (61, -41)
  line L4 (61, -41) -> (67.5, -41)
  line L5 (67.5, -41) -> (67.5, 41)
  line L6 (67.5, 41) -> (38.5, 41)
  line L7 (-67.5, 41) -> (-67.5, -41)
  line L8 (-67.5, -41) -> (-25, -41)
  line L9 (-25, -41) -> (-25, -16)
  line L10 (-25, -16) -> (0.5, -16)
  line L11 (38.5, 33) -> (32.5, 33)
  line L12 (32.5, 33) -> (32.5, 41)
  line L13 (38.5, 41) -> (38.5, 33)
  line L14 (-38.5, -5) -> (-32.5, -5)
  line L15 (-32.5, -5) -> (-32.5, -11)
  line L16 (-38.5, -11) -> (-38.5, -5)
  line L17 (-67.5, 19) -> (-57.5, 19)
  line L18 (-57.5, 19) -> (-57.5, -11)
  line L19 (-57.5, -11) -> (-67.5, -11)
  line L20 (-67.5, -11) -> (-67.5, 19)
  line L21 (-69, 35.25) -> (-67.5, 35.25)
  line L22 (-67.5, 35.25) -> (-67.5, 41)
  line L23 (-67.5, 41) -> (67.5, 41)
  line L24 (67.5, 41) -> (67.5, 2)
  line L25 (67.5, 2) -> (69, 2)
  line L26 (69, 2) -> (69, 42.5)
  line L27 (69, 42.5) -> (-69, 42.5)
  line L28 (-69, 42.5) -> (-69, 35.25)
  line L29 (-38.5, 35) -> (-38.5, 41)
  line L30 (-34.5, 41) -> (-34.5, 35)
  line L31 (-34.5, 35) -> (-38.5, 35)
  line L32 (38.5, -7) -> (38.5, -16)
  line L33 (34.5, -11) -> (34.5, -7)
  line L34 (34.5, -7) -> (38.5, -7)
  line L35 (38.5, -16) -> (61, -16)
  line L36 (32.5, 41) -> (-34.5, 41)
  line L37 (-38.5, 41) -> (-67.5, 41)
  line L38 (35.5, -11) -> (34.5, -11)
  line L39 (-32.5, -11) -> (-38.5, -11)
  dimension "d175" = 10
  dimension "d176" = 30
  dimension "d179" = 22
  constraint horizontal L17
  constraint vertical L18
  constraint horizontal L19
  constraint vertical L20
  constraint coincident L7 L17.start
  measures "d175" distance of L17.start L17.end
  measures "d176" distance of L17.start L19.end
  measures "d179" distance of L17 L23
extrude "Extrusion28" add sketch "Skizze23" along normal blind 30 separate body contours L7 L17 L18 L19 L20 makes body 3
sketch "Skizze25" plane through (69, 0, 0) normal (1, 0, 0) x (0, 0, -1)
  line L0 (42.5, 32.5) -> (-42.5, 32.5)
  line L1 (-42.5, 32.5) -> (-42.5, 14)
  line L2 (-42.5, 14) -> (-35.25, 14)
  arc A0 (-26.75, 14) -> (-35.25, 14) centre (-31, 14) ccw
  line L3 (-26.75, 14) -> (23, 14)
  arc A1 (32, 14) -> (23, 14) centre (27.5, 14) ccw
  line L4 (32, 14) -> (42.5, 14)
  line L5 (42.5, 14) -> (42.5, 32.5)
  line L6 (11, 1.5) -> (-19, 1.5)
  line L7 (-19, 1.5) -> (-19, 31.5)
  line L8 (-19, 31.5) -> (11, 31.5)
  line L9 (11, 31.5) -> (11, 1.5)
  line L10 (-19, 31.5) -> (11, 1.5)
  line L11 (-19, 1.5) -> (11, 31.5)
  circle A2 centre (-4, 16.5) radius 14.5
  dimension "d180" = 29
  constraint coincident L7.end L8.start
  constraint coincident L6.start L9.end
  constraint coincident L6.end L7.start
  constraint coincident L8.end L9.start
  constraint midpoint L10 A2.centre
  measures "d180" diameter of A2
extrude "Extrusion29" cut sketch "Skizze25" against normal blind 1.5 contours L3 L10 A2 | L3 L11 A2 | L3 L10 L11 A2 picked at (-3.6552, 10.0123) bodies 1
sketch "Skizze27" plane through (67.5, 0, 0) normal (1, 0, 0) x (0, 0, -1)
  line L0 (-19, 1.5) -> (11, 1.5)
  line L1 (11, 1.5) -> (11, 31.5)
  line L2 (11, 31.5) -> (-19, 31.5)
  line L3 (-19, 31.5) -> (-19, 1.5)
  line L4 (-19, 31.5) -> (11, 1.5)
  line L5 (-19, 1.5) -> (11, 31.5)
  circle A0 centre (-4, 16.5) radius 14.5
  dimension "d183" = 29
  constraint coincident L2.end L3.start
  constraint coincident L0.end L1.start
  constraint coincident L0.start L3.end
  constraint coincident L1.end L2.start
  constraint midpoint L4 A0.centre
  measures "d183" diameter of A0
extrude "Extrusion30" cut sketch "Skizze27" against normal blind 10 contours L4 L5 A0 | L4 L5 A0 | L4 L5 A0 | L4 L5 A0 bodies 3
sketch "Skizze28" plane through (69, 0, 0) normal (1, 0, 0) x (0, 0, -1)
  line L0 (42.5, 32.5) -> (-42.5, 32.5)
  line L1 (-42.5, 32.5) -> (-42.5, 14)
  line L2 (-42.5, 14) -> (-35.25, 14)
  arc A0 (-26.75, 14) -> (-35.25, 14) centre (-31, 14) ccw
  line L3 (-26.75, 14) -> (23, 14)
  arc A1 (32, 14) -> (23, 14) centre (27.5, 14) ccw
  line L4 (32, 14) -> (42.5, 14)
  line L5 (42.5, 14) -> (42.5, 32.5)
  circle A2 centre (-4, 16.5) radius 14.5
  line L6 (-19, 1.5) -> (11, 1.5)
  line L7 (11, 1.5) -> (11, 31.5)
  line L8 (11, 31.5) -> (-19, 31.5)
  line L9 (-19, 31.5) -> (-19, 1.5)
  circle A3 centre (-4, 16.5) radius 14
  constraint concentric A2 A3